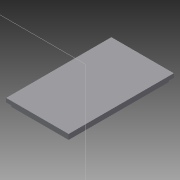
# Autodesk Inventor part: Transmitter Case Top
Saved by Autodesk Inventor 2014 SP1 (Build 180222100, 222)
## iProperties
Created: 2014-05-14
Part Number: Transmitter Case Top
Material: Generic
Document SubType Name: Modeling
Designer: Alex
Density: 1 g/cm^3
Appearance: Default
Author: Alex
Autodesk Inventor part; units mm, degrees
ref_plane "YZ Plane" through (0, 0, 0) normal (1, 0, 0) x (0, 1, 0)
ref_plane "XZ Plane" through (0, 0, 0) normal (0, 1, 0) x (-1, 0, 0)
ref_plane "XY Plane" through (0, 0, 0) normal (0, 0, 1) x (1, 0, 0)
sketch "Sketch1" plane through (0, 0, 0) normal (0, 0, 1) x (1, 0, 0)
  line L0 (0, 0) -> (45, 0)
  line L1 (45, 0) -> (45, 78.5)
  line L2 (45, 78.5) -> (0, 78.5)
  line L3 (0, 78.5) -> (0, 0)
  dimension "d0" = 45
  dimension "d1" = 78.5
  constraints: 8 end point, 2 parallel, 1 horizontal, 1 perpendicular
  measures "d0" distance of L2.end L1.end
  measures "d1" distance of L1.end L0.end
extrude "Extrusion1" add sketch "Sketch1" along normal blind 3
sketch "Sketch2" plane through (0, 0, 3) normal (0, 0, 1) x (1, 0, 0)
  line L0 (0, 78.5) -> (-2, 78.5)
  line L1 (-2, 78.5) -> (-2, 80.5)
  line L2 (-2, 80.5) -> (0, 80.5)
  line L3 (0, 80.5) -> (0, 78.5)
  line L4 (45, 0) -> (47, 0)
  line L5 (47, 0) -> (47, -2)
  line L6 (47, -2) -> (45, -2)
  line L7 (45, -2) -> (45, 0)
  line L8 (-2, 80.5) -> (47, 80.5)
  line L9 (47, 80.5) -> (47, -2)
  line L10 (47, -2) -> (-2, -2)
  line L11 (-2, -2) -> (-2, 80.5)
  dimension "d4" = 2
  dimension "d5" = 2
  dimension "d6" = 2
  dimension "d7" = 2
  constraints: 24 end point, 6 parallel, 3 horizontal, 3 perpendicular
  measures "d4" distance of L1.end L2.end
  measures "d5" distance of L0.end L1.end
  measures "d6" distance of L5.end L6.end
  measures "d7" distance of L4.end L5.end
extrude "Extrusion2" add sketch "Sketch2" along normal blind 3
body "Solid1"
